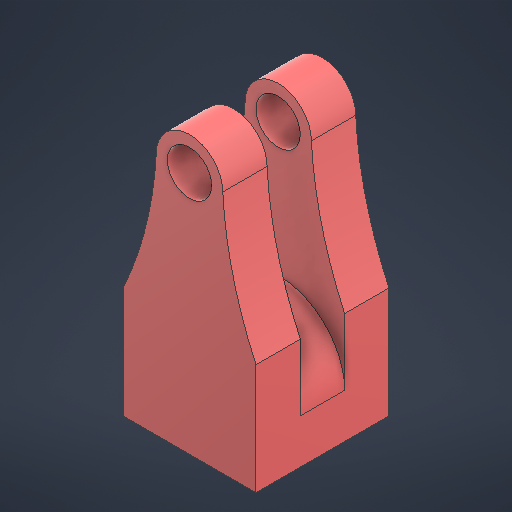
# Autodesk Inventor part: Connector_hollow
Saved by Autodesk Inventor 2027 (Build 310192060, 192F)
## iProperties
Created: 2026-08-01
Part Number: Connector_hollow
Material: Ogólny
Document SubType Name: Modeling
Designer: User
Density: 1 g/cm^3
Appearance: Domyślna
Author: User
Autodesk Inventor part; units mm, degrees
ref_plane "YZ Plane" through (0, 0, 0) normal (1, 0, 0) x (0, 1, 0)
sketch "Szkic3" plane through (0, 0, 0) normal (0, 1, 0) x (-1, 0, 0)
  circle A0 centre (0, 0) radius 5
  line L0 (-6, -6) -> (6, -6)
  line L1 (6, -6) -> (6, 6)
  line L2 (6, 6) -> (-6, 6)
  line L3 (-6, 6) -> (-6, -6)
  line L4 (-6, -6) -> (6, 6) construction
  line L5 (6, -6) -> (-6, 6) construction
  dimension "d12" = 10
  dimension "d15" = 12
  dimension "d16" = 12
  constraints: 12 end point, 2 midpoint, 2 parallel, 1 centre point, 1 coincident, 1 horizontal, 1 perpendicular
  measures "d12" diameter of A0
  measures "d15" distance of L2.end L1.end
  measures "d16" distance of L1.end L0.end
extrude "Wyciągnięcie proste3" add sketch "Szkic3" along normal mid plane 10
extrude "Wyciągnięcie proste4" add sketch "Szkic3" along normal blind 5 contours A0
ref_plane "Płaszczyzna konstrukcyjna2" through (-6, 5, 0) normal (0, 0, 1) x (1, 0, 0)
sketch "Szkic7" plane through (-6, 5, 0) normal (0, 0, 1) x (1, 0, 0)
  line L0 (0, -10) -> (0, 0) projected
  line L1 (0, 0) -> (12, 0)
  line L2 (12, 0) -> (6, 0)
  line L3 (6, 0) -> (6, 12) construction
  circle A0 centre (6, 12) radius 2
  line L4 (6, 12) -> (8, 12) construction
  line L5 (8, 12) -> (9, 12)
  line L6 (6, 12) -> (6, 14) construction
  line L7 (6, 14) -> (6, 15)
  arc A1 (9, 12) -> (6, 15) centre (6, 12) ccw
  arc A2 (9, 12) -> (12, 0) centre (41.9474, 13.8619) ccw
  line L8 (4, 12) -> (3, 12)
  arc A3 (6, 15) -> (3, 12) centre (6, 12) ccw
  arc A4 (0, 0) -> (3, 12) centre (-29.9474, 13.8619) ccw
  point P0 (6, -5)
  dimension "d61" = 12
  dimension "d62" = 4
  dimension "d63" = 1
  dimension "d64" = 2
  dimension "d65" = 1
  dimension "d66" = 3
  dimension "d67" = 33
  dimension "d68" = 1
  dimension "d69" = 2
  dimension "d70" = 3
  dimension "d71" = 33
  constraints: 16 end point, 11 point on circle, 5 centre point, 3 horizontal, 3 vertical, 1 coincident, 1 midpoint, 1 point on line
  measures "d61" distance of L2.end L3.end
  measures "d62" diameter of A0
  measures "d63" distance of L4.end L5.end
  measures "d64" distance of L3.end L4.end
  measures "d65" distance of L6.end L7.end
  measures "d66" radius of A1
  measures "d67" radius of A2
  measures "d68" distance of L8.start L8.end
  measures "d69" distance of L4.start L8.start
  measures "d70" radius of A3
  measures "d71" radius of A4
extrude "Wyciągnięcie proste7" add sketch "Szkic7" along normal mid plane 12 contours A4 L8 A0 L5 A2 L1 | A3 L7 A0 L8 | A1 L5 A0 L7
ref_plane "Płaszczyzna konstrukcyjna3" through (-6, -5, 0) normal (0, 0, 1) x (1, 0, 0)
sketch "Szkic9" plane through (-6, -5, 0) normal (0, 0, 1) x (1, 0, 0)
  arc A0 (9, 22) -> (12, 10) centre (41.9474, 23.8619) ccw projected
  line L0 (0, 34) -> (12, 34)
  line L1 (12, 34) -> (12, 10)
  line L2 (12, 10) -> (0, 10)
  line L3 (0, 10) -> (0, 34)
  circle A1 centre (6, 22) radius 2 projected
  line L4 (0, 34) -> (12, 10) construction
  line L5 (12, 34) -> (0, 10) construction
  point P0 (6, 5)
  constraints: 12 end point, 2 midpoint, 2 parallel, 1 horizontal, 1 perpendicular
extrude "Wyciągnięcie proste9" cut sketch "Szkic9" along normal mid plane 4
fillet "Zaokrąglenie7" radius 6 2 edges at (6, 5, 0) (-6, 5, 0)
